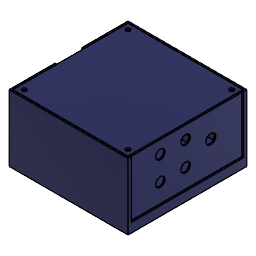
Matching box (Autodesk Fusion 360 design; units mm, degrees)
part number: 2026-08-06-16-31-01-128
Autodesk Fusion 360 part; units mm, degrees
note: some values were not read from the file. Set by a fixed rule: which face or edge a step refers to.
sketch "Sketch1" plane through (0, 0, 0) normal (0, 0, 1) x (1, 0, 0)
  line L0 (42.25, -42.25) -> (-42.25, -42.25)
  line L1 (-42.25, -42.25) -> (-42.25, 42.25)
  line L2 (-42.25, 42.25) -> (42.25, 42.25)
  line L3 (42.25, 42.25) -> (42.25, -42.25)
  line L4 (42.25, -42.25) -> (-42.25, 42.25) construction
  line L5 (-42.25, -42.25) -> (42.25, 42.25) construction
  line L6 (44.75, -44.75) -> (-44.75, -44.75)
  line L7 (-44.75, -44.75) -> (-44.75, 44.75)
  line L8 (-44.75, 44.75) -> (44.75, 44.75)
  line L9 (44.75, 44.75) -> (44.75, -44.75)
  line L10 (44.75, -44.75) -> (-44.75, 44.75) construction
  line L11 (-44.75, -44.75) -> (44.75, 44.75) construction
  line L12 (44.75, -42.25) -> (42.25, -42.25)
  line L13 (42.25, 42.25) -> (44.75, 42.25)
  line L14 (43.5, -42.25) -> (43.5, -43.5)
  line L15 (42.25, -43.5) -> (42.25, -42.25)
  line L16 (43.5, -43.5) -> (42.25, -43.5)
  line L17 (44.75, 0) -> (-44.75, 0)
  circle A0 centre (25.4, -25.4) radius 0.5
  line L18 (0, -44.75) -> (0, 44.75)
  circle A1 centre (25.4, -25.4) radius 2.5
  circle A2 centre (25.4, 25.4) radius 2.5
  circle A3 centre (25.4, 25.4) radius 0.5
  line L19 (25.4, -25.4) -> (25.4, 25.4) construction
  circle A4 centre (-25.4, -25.4) radius 2.5
  circle A5 centre (-25.4, -25.4) radius 0.5
  circle A6 centre (-25.4, 25.4) radius 2.5
  circle A7 centre (-25.4, 25.4) radius 0.5
  line L20 (43.5, 43.5) -> (42.25, 43.5)
  line L21 (43.5, 42.25) -> (43.5, 43.5)
  line L22 (42.25, 43.5) -> (42.25, 42.25)
  line L23 (-44.75, 10) -> (-42.25, 10)
  line L24 (-44.75, -10) -> (-42.25, -10)
  line L25 (43.5, 42.25) -> (43.5, -42.25)
  line L26 (35.75, -35.75) -> (-35.75, -35.75)
  line L27 (-35.75, -35.75) -> (-35.75, 35.75)
  line L28 (-35.75, 35.75) -> (35.75, 35.75)
  line L29 (35.75, 35.75) -> (35.75, -35.75)
  line L30 (35.75, -35.75) -> (-35.75, 35.75) construction
  line L31 (-35.75, -35.75) -> (35.75, 35.75) construction
  line L32 (42.25, -43.5) -> (-43.5, -43.5)
  line L33 (-43.5, -43.5) -> (-43.5, 43.5)
  line L34 (-43.5, 43.5) -> (42.25, 43.5)
  line L35 (-35.75, -35.75) -> (-35.75, -42.25)
  line L36 (-35.75, -35.75) -> (-42.25, -35.75)
  circle A8 centre (-39, -39) radius 2
  line L37 (-39, -42.25) -> (-39, -35.75) construction
  line L38 (35.75, -35.75) -> (42.25, -35.75)
  line L39 (35.75, -35.75) -> (35.75, -42.25)
  circle A9 centre (39, -39) radius 2
  circle A10 centre (-39, 39) radius 2
  line L40 (-35.75, 35.75) -> (-42.25, 35.75)
  line L41 (-35.75, 35.75) -> (-35.75, 42.25)
  circle A11 centre (39, 39) radius 2
  line L42 (35.75, 35.75) -> (35.75, 42.25)
  line L43 (35.75, 35.75) -> (42.25, 35.75)
  circle A12 centre (-39, -39) radius 1.625
  circle A13 centre (39, -39) radius 1.625
  circle A14 centre (-39, 39) radius 1.625
  circle A15 centre (39, 39) radius 1.625
  dimension "d2" = 84.5
  dimension "d3" = 2.5
  dimension "d6" = 1
  dimension "d7" = 5
  dimension "d9" = 50.8
  dimension "d15" = 20
  dimension "d35" = 6.5
  dimension "d46" = 4
  dimension "d52" = 3.25
  constraint horizontal L0
  constraint perpendicular L0 L1
  constraint parallel L0 L2
  constraint parallel L1 L3
  constraint coincident L4 origin
  constraint coincident L5 origin
  constraint equal L0 L1
  constraint horizontal L6
  constraint perpendicular L6 L7
  constraint parallel L6 L8
  constraint parallel L7 L9
  constraint coincident L10 origin
  constraint coincident L11 origin
  constraint equal L6 L7
  constraint coincident L9 L12.start
  constraint perpendicular L3 L12
  constraint coincident L9 L13.end
  constraint perpendicular L9 L13
  constraint midpoint L12 L14.start
  constraint coincident L10 L14.end
  constraint perpendicular L12 L14
  constraint perpendicular L14 L16
  constraint vertical L15
  constraint horizontal L17
  constraint coincident origin L17
  constraint coincident L10 A0.centre
  constraint perpendicular L8 L18
  constraint midpoint L6 L18.start
  constraint midpoint L8 L18.end
  constraint midpoint L9 L17.start
  constraint midpoint L7 L17.end
  constraint concentric A0 A1
  constraint symmetric L17 A0 A3
  constraint symmetric L17 A1 A2
  constraint coincident A0.centre A1.centre
  constraint coincident A2.centre A3.centre
  constraint symmetric A0 L18 A5
  constraint symmetric L18 A1 A4
  constraint symmetric L18 A2 A6
  constraint symmetric L18 A3 A7
  constraint symmetric L0.start L17 L2.end
  constraint symmetric L14.start L17 L21.start
  constraint symmetric L14.end L17 L20.start
  constraint symmetric L15.start L17 L20.end
  constraint coincident L7 L23.start
  constraint coincident L1 L23.end
  constraint perpendicular L1 L23
  constraint symmetric L17 L23.start L24.start
  constraint symmetric L17 L23.end L24.end
  constraint horizontal L26
  constraint perpendicular L26 L27
  constraint parallel L26 L28
  constraint parallel L27 L29
  constraint coincident L30 origin
  constraint coincident L31 origin
  constraint equal L26 L27
  constraint coincident L11 L32.end
  constraint perpendicular L15 L32
  constraint coincident L10 L33.end
  constraint perpendicular L32 L33
  constraint coincident L0 L35.end
  constraint perpendicular L0 L35
  constraint coincident L1 L36.end
  constraint perpendicular L1 L36
  constraint coincident L11 A8.centre
  constraint coincident L0 L37.start
  constraint midpoint L36 L37.end
  constraint midpoint A8.centre L37
  constraint symmetric L18 L26.end L26.start
  constraint symmetric L18 L35.end L39.end
  constraint symmetric L18 L36.end L38.end
  constraint symmetric L18 A8 A9
  constraint symmetric L17 L26.end L27.end
  constraint symmetric L17 L35.end L41.end
  constraint symmetric L17 L36.end L40.end
  constraint symmetric L17 A8 A10
  constraint symmetric L17 L26.start L28.end
  constraint symmetric L17 L38.end L43.end
  constraint symmetric L17 L39.end L42.end
  constraint symmetric L17 A9 A11
  constraint concentric A8 A12
  constraint symmetric L18 A12 A13
  constraint symmetric L17 A12 A14
  constraint symmetric L17 A13 A15
  measures "d2" distance of L0.start L0.end
  measures "d3" distance of L0 L6
  measures "d6" diameter of A0
  measures "d7" diameter of A1
  measures "d9" distance of A0.centre A2.centre
  measures "d35" distance of L0 L26
  measures "d46" diameter of A8
  measures "d52" diameter of A12
extrude "Extrude1" add sketch "Sketch1" along normal blind 2 contours L0 L15 L18 L32 | L0 L3 L38 L39 | L3 L12 L17 L25 | L12 L14 L15 L16 | L0 L18 L26 L39 | L3 L17 L29 L38 | L9 L12 L17 L25 | L6 L9 L12 L14 L16 L18 L32 | L0 L1 L18 L24 L32 L33 | L0 L18 L26 L35 | L17 L18 L26 L29 | L3 L17 L29 L43 | L3 L13 L17 L25 | L9 L13 L17 L25 | L6 L7 L18 L24 L32 L33 | L0 L1 L35 L36 | L17 L18 L26 L27 | L17 L18 L28 L29 | L2 L3 L42 L43 | L8 L9 L13 L18 L20 L21 L34 | L13 L20 L21 L22 | L1 L17 L27 L36 | L17 L18 L27 L28 | L2 L18 L28 L42 | L2 L18 L22 L34 | L1 L17 L24 L33 | L7 L17 L24 L33 | L1 L17 L27 L40 | L2 L18 L28 L41 | L1 L17 L23 L33 | L7 L17 L23 L33 | L1 L2 L40 L41 | L1 L2 L18 L23 L33 L34 | L7 L8 L18 L23 L33 L34 | A0 | A1 | A2 | A3 | A4 | A5 | A6 | A7 | A8 | A9 | A10 | A11 | A12 | A13 | A14 | A15 makes body 1
extrude "Extrude2" add sketch "Sketch1" along normal blind 48 from surface at 2 contours L0 L15 L18 L32 | L0 L3 L38 L39 | L6 L9 L12 L14 L16 L18 L32 | L0 L1 L18 L24 L32 L33 | L6 L7 L18 L24 L32 L33 | L0 L1 L35 L36 | L2 L3 L42 L43 | L8 L9 L13 L18 L20 L21 L34 | L2 L18 L22 L34 | L1 L2 L40 L41 | L1 L2 L18 L23 L33 L34 | L7 L8 L18 L23 L33 L34 bodies 1
extrude "Extrude3" add sketch "Sketch1" along normal blind 5 from surface at 2 contours L0 L3 L38 L39 | L0 L18 L26 L39 | L3 L17 L29 L38 | L9 L12 L17 L25 | L0 L18 L26 L35 | L3 L17 L29 L43 | L9 L13 L17 L25 | L0 L1 L35 L36 | L2 L3 L42 L43 | L1 L17 L27 L36 | L2 L18 L28 L42 | L1 L17 L24 L33 | L7 L17 L24 L33 | L1 L17 L27 L40 | L2 L18 L28 L41 | L1 L17 L23 L33 | L7 L17 L23 L33 | L1 L2 L40 L41 | A0 | A1 | A2 | A3 | A4 | A5 | A6 | A7 | A8 | A9 | A10 | A11 | A12 | A13 | A14 | A15 bodies 1
extrude "Extrude4" add sketch "Sketch1" along normal blind 3 from surface at 7 contours L1 L17 L24 L33 | L7 L17 L24 L33 | L1 L17 L23 L33 | L7 L17 L23 L33 | A0 | A3 | A5 | A7 bodies 1
extrude "Extrude6" add sketch "Sketch1" along normal up to surface (48 mm away) from surface at 2 separate body contours L3 L12 L17 L25 | L12 L14 L15 L16 | L3 L13 L17 L25 | L13 L20 L21 L22 makes body 2
move_face "OffsetFaces3" offset -0.15 5 faces at (43.5, -14.0833, 18) (43.0833, 43.5, 18) (42.25, 23.8333, 18) (43.0833, 26, 2) (43.0833, -43.5, 18) on bodies 2
sketch "Sketch4" plane through (-42.25, 0, 0) normal (1, 0, 0) x (0, 1, 0)
  line L0 (-35.75, 7) -> (35.75, 7)
  line L1 (35.75, 50) -> (10, 50)
  line L2 (10, 50) -> (10, 10)
  line L3 (10, 10) -> (-10, 10)
  line L4 (-10, 10) -> (-10, 50)
  circle A0 centre (0, 39) radius 3.5
  line L5 (0, 0) -> (0, 50.8856) construction
  line L6 (-39.802, 30) -> (50, 30) construction
  line L7 (35.75, 7) -> (35.75, 50)
  line L8 (-10, 50) -> (-35.75, 50)
  line L9 (-35.75, 50) -> (-35.75, 7)
  circle A1 centre (0, 21) radius 3.5
  circle A2 centre (19, 30) radius 3.7175
  circle A3 centre (-19, 39) radius 3.5
  circle A4 centre (-19, 21) radius 3.5
  dimension "d41" = 7
  dimension "d44" = 30
  dimension "d57" = 9
  dimension "d61" = 19
  dimension "d62" = 7
  dimension "d63" = 19
  constraint coincident L5.start origin
  constraint perpendicular L0 L5
  constraint horizontal L6
  constraint symmetric A0 L6 A1
  constraint coincident L6 A2.centre
  constraint coincident A0.centre L5
  constraint symmetric L6 A3 A4
  measures "d41" diameter of A0
  measures "d44" distance of L5.start L6
  measures "d57" distance of A0.centre L6
  measures "d61" distance of L5 A2.centre
  measures "d62" diameter of A3
  measures "d63" distance of L5 A3.centre
extrude "Extrude7" cut sketch "Sketch4" along normal up to surface (0.95 mm away) from surface at 84.65 contours A0 | A1 | A2 | A3 | A4 bodies 2
extrude "Extrude8" cut sketch "Sketch1" against normal blind 1.25 from surface at 50 contours L0 L15 L18 L32 | L0 L3 L38 L39 | L3 L12 L17 L25 | L12 L14 L15 L16 | L0 L1 L18 L24 L32 L33 | L3 L13 L17 L25 | L0 L1 L35 L36 | L2 L3 L42 L43 | L13 L20 L21 L22 | L2 L18 L22 L34 | L1 L2 L40 L41 | L1 L2 L18 L23 L33 L34 bodies 1 2
fillet "Fillet1" radius 1 4 edges at (-35.75, 35.75, 27.875) (-35.75, -35.75, 27.875) (35.75, 35.75, 27.875) (35.75, -35.75, 27.875) on bodies 1
extrude "Extrude9" add sketch "Sketch1" along normal up to surface (1.25 mm away) from surface at 48.75 separate body contours L0 L15 L18 L32 | L0 L3 L38 L39 | L3 L12 L17 L25 | L12 L14 L15 L16 | L0 L18 L26 L39 | L3 L17 L29 L38 | L0 L1 L18 L24 L32 L33 | L0 L18 L26 L35 | L17 L18 L26 L29 | L3 L17 L29 L43 | L3 L13 L17 L25 | L0 L1 L35 L36 | L17 L18 L26 L27 | L17 L18 L28 L29 | L2 L3 L42 L43 | L13 L20 L21 L22 | L1 L17 L27 L36 | L17 L18 L27 L28 | L2 L18 L28 L42 | L2 L18 L22 L34 | L1 L17 L24 L33 | L1 L17 L27 L40 | L2 L18 L28 L41 | L1 L17 L23 L33 | L1 L2 L40 L41 | L1 L2 L18 L23 L33 L34 | A0 | A1 | A2 | A3 | A4 | A5 | A6 | A7 | A8 | A9 | A10 | A11 makes body 3
move_face "OffsetFaces4" offset -0.15 4 faces at (43.5, -14.0833, 49.1667) (43.0833, 43.5, 49.1667) (-43.5, -32.3333, 49.5833) (-14.5, -43.5, 49.1667) on bodies 3
equation "d9 = 2.54 * 20 mm"
named bodies: "Matching box", "Matching box front panel", "Matching box lid"
